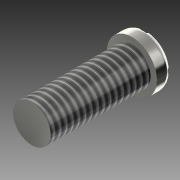
# Autodesk Inventor part: 8mm M3
Saved by Autodesk Inventor 2015 (Build 190159000, 159)
## iProperties
Created: 2016-10-18
Part Number: 8mm M3
Material: Generic
Document SubType Name: Modeling
Designer: James Yelland
Density: 1 g/cm^3
Appearance: Silver
Author: James Yelland
Autodesk Inventor part; units mm, degrees
ref_plane "YZ Plane" through (0, 0, 0) normal (1, 0, 0) x (0, 1, 0)
ref_plane "XZ Plane" through (0, 0, 0) normal (0, 1, 0) x (-1, 0, 0)
ref_plane "XY Plane" through (0, 0, 0) normal (0, 0, 1) x (1, 0, 0)
sketch "Sketch1" plane through (0, 0, 0) normal (0, 1, 0) x (-1, 0, 0)
  circle A0 centre (0, 0) radius 1.5
  dimension "d0" = 3
  constraints: 1 centre point, 1 coincident
  measures "d0" diameter of A0
extrude "Extrusion1" add sketch "Sketch1" along normal blind 8
sketch "Sketch2" plane through (0, 8, 0) normal (0, 1, 0) x (1, 0, 0)
  circle A0 centre (0, 0) radius 2
  dimension "d3" = 4
  constraints: 1 centre point, 1 coincident
  measures "d3" diameter of A0
extrude "Extrusion2" add sketch "Sketch2" along normal blind 1.3
fillet "Fillet1" radius 0.6 1 edges at (-2, 9.3, 0)
thread "Thread1" size "M3x0.5" class "6g" standard "ANSI Metric M Profile" full length
sketch "Sketch3" plane through (0, 9.3, 0) normal (0, 1, 0) x (1, 0, 0)
  line L0 (0.25, 2.5) -> (-0.25, 2.5)
  line L1 (-0.25, 2.5) -> (-0.25, -2.5)
  line L2 (-0.25, -2.5) -> (0.25, -2.5)
  line L3 (0.25, -2.5) -> (0.25, 2.5)
  line L4 (0.25, 2.5) -> (-0.25, -2.5) construction
  line L5 (-0.25, 2.5) -> (0.25, -2.5) construction
  line L6 (2.5, 0.25) -> (2.5, -0.25)
  line L7 (2.5, -0.25) -> (-2.5, -0.25)
  line L8 (-2.5, -0.25) -> (-2.5, 0.25)
  line L9 (-2.5, 0.25) -> (2.5, 0.25)
  line L10 (2.5, 0.25) -> (-2.5, -0.25) construction
  line L11 (2.5, -0.25) -> (-2.5, 0.25) construction
  line L12 (2.5, 0.25) -> (3, 0.25) construction
  point P0 (0, 0)
  dimension "d9" = 0.5
  dimension "d10" = 5
  dimension "d11" = 0.5
  dimension "d12" = 90
  dimension "d13" = 5
  constraints: 26 end point, 5 parallel, 4 midpoint, 3 perpendicular, 2 horizontal
  measures "d9" distance of L0.start L0.end
  measures "d10" distance of L1.end L0.end
  measures "d11" distance of L6.start L6.end
  measures "d12" angle of L6 L12
  measures "d13" distance of L6.end L7.end
extrude "Extrusion3" cut sketch "Sketch3" against normal blind 0.4
body "Solid1"
